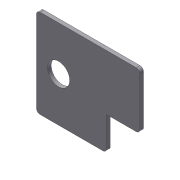
# Autodesk Inventor part: Plate_VerticalRollerMount_Top
Saved by Autodesk Inventor 2012 (Build 160160000, 160)
## iProperties
Created: 2012-01-21
Part Number: Plate_VerticalRollerMount_Top
Material: Aluminum-6061
Document SubType Name: Modeling
Designer: JesseK
Mass: 48.7156 g
Surface Area: 125.404 cm^2
Volume: 17.9762 cm^3
Density: 2.71 g/cm^3
Author: JesseK
Autodesk Inventor part; units mm, degrees
ref_plane "YZ Plane" through (0, 0, 0) normal (1, 0, 0) x (0, 1, 0)
ref_plane "XZ Plane" through (0, 0, 0) normal (0, 1, 0) x (-1, 0, 0)
ref_plane "XY Plane" through (0, 0, 0) normal (0, 0, 1) x (1, 0, 0)
sketch "Sketch1" plane through (0, 0, 0) normal (0, 0, 1) x (1, 0, 0)
  line L0 (0, 0) -> (88.9, 0)
  line L1 (88.9, 0) -> (88.9, 76.2)
  line L2 (88.9, 76.2) -> (0, 76.2)
  line L3 (0, 76.2) -> (0, 0)
  dimension "d9" = 88.9
  dimension "d10" = 76.2
  constraints: 8 end point, 2 parallel, 1 coincident, 1 horizontal, 1 perpendicular
  measures "d9" distance between parallel lines of L1 L3
  measures "d10" distance between parallel lines of L0 L2
extrude "Extrusion1" add sketch "Sketch1" along normal blind 3.175
sketch "Sketch3" plane through (0, 0, 3.175) normal (0, 0, 1) x (1, 0, 0)
  line L0 (88.9, 0) -> (60.325, 0)
  line L1 (60.325, 0) -> (60.325, 28.575)
  line L2 (60.325, 28.575) -> (88.9, 28.575)
  line L3 (88.9, 28.575) -> (88.9, 0)
  dimension "d12" = 28.575
  constraints: 8 end point, 2 parallel, 2 perpendicular, 1 horizontal
  measures "d12" distance of L1.end L2.end
extrude "Extrusion3" cut sketch "Sketch3" against normal through all
sketch "Sketch4" plane through (0, 0, 3.175) normal (0, 0, 1) x (1, 0, 0)
  line L0 (0, 0) -> (0, 76.2) projected
  line L1 (60.325, 0) -> (0, 0) projected
  circle A0 centre (19.05, 38.1) radius 9.525
  dimension "d15" = 19.05
  dimension "d16" = 38.1
  dimension "d17" = 19.05
  constraints: 1 centre point
  measures "d15" diameter of A0
  measures "d16" distance from line of L1 A0.centre
  measures "d17" distance from line of L0 A0.centre
extrude "Extrusion4" cut sketch "Sketch4" against normal through all
fillet "Fillet1" radius 3.175 5 edges at (0, 76.2, 1.5875) (0, 0, 1.5875) (60.325, 0, 1.5875) (88.9, 28.575, 1.5875) (88.9, 76.2, 1.5875)
body "Solid1"
